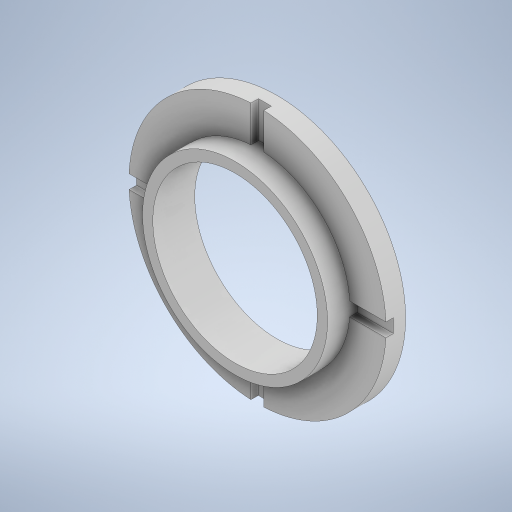
# Autodesk Inventor part: KY 58 Part
Saved by Autodesk Inventor 2024 (Build 280153000, 153)
## iProperties
Created: 2024-12-26
Part Number: KY 58 Part
Material: Generic
Document SubType Name: Modeling
Designer: Administrator
Density: 1 g/cm^3
Appearance: Default
Author: Administrator
Autodesk Inventor part; units mm, degrees
ref_plane "YZ Plane" through (0, 0, 0) normal (1, 0, 0) x (0, 1, 0)
ref_plane "XZ Plane" through (0, 0, 0) normal (0, 1, 0) x (-1, 0, 0)
ref_plane "XY Plane" through (0, 0, 0) normal (0, 0, 1) x (1, 0, 0)
sketch "Sketch1" plane through (0, 0, 0) normal (0, 0, 1) x (1, 0, 0)
  line L0 (-73.2799, 44.0426) -> (79.8189, 44.0426) construction
  line L1 (79.8189, 44.0426) -> (79.8189, -42.434) construction
  line L2 (79.8189, -42.434) -> (-73.2799, -42.434) construction
  line L3 (-73.2799, -42.434) -> (-73.2799, 44.0426) construction
  circle A0 centre (0.9241, -2.5998) radius 8.239
  circle A1 centre (0.9241, -2.5998) radius 12.8881
  point P0 (0, 0)
  constraints: 2 centre point, 2 other
extrude "Extrusion1" add sketch "Sketch1" along normal blind 1.2
sketch "Sketch2" plane through (0.9241, -2.5998, 1.2) normal (0, 0, 1) x (1, 0, 0)
  circle A0 centre (0, 0) radius 8.239 projected
  circle A1 centre (0, 0) radius 9.2643
  point P0 (-0.9241, 2.5998)
  constraints: 1 centre point
extrude "Extrusion2" add sketch "Sketch2" along normal blind 3
sketch "Sketch3" plane through (0.9241, -2.5998, 1.2) normal (0, 0, 1) x (1, 0, 0)
  circle A0 centre (0, 0) radius 9.1906
  arc A1 (12.8725, 0.6343) -> (0.6367, 12.8724) centre (0, 0) ccw
  arc A2 (-0.6581, 12.8713) -> (-12.8725, 0.6343) centre (0, 0) ccw
  arc A3 (-12.8667, -0.7427) -> (-0.6581, -12.8713) centre (0, 0) ccw
  arc A4 (0.6367, -12.8724) -> (12.8667, -0.7427) centre (0, 0) ccw
  line L0 (-12.8725, 0.6343) -> (-9.1687, 0.6343)
  line L1 (-9.1605, -0.7427) -> (-12.8667, -0.7427)
  line L2 (-0.6581, -12.8713) -> (-0.6581, -9.167)
  line L3 (0.6367, -9.1685) -> (0.6367, -12.8724)
  line L4 (12.8667, -0.7427) -> (9.1605, -0.7427)
  line L5 (9.1687, 0.6343) -> (12.8725, 0.6343)
  line L6 (0.6367, 12.8724) -> (0.6367, 9.1685)
  line L7 (-0.6581, 9.167) -> (-0.6581, 12.8713)
  point P0 (-0.9241, 2.5998)
  constraints: 16 end point, 8 parallel, 8 point on circle, 4 centre point, 1 coincident, 10 other
extrude "Extrusion3" add sketch "Sketch3" along normal blind 0.75 contours A0 L6 A1 L5 | L4 A4 L3 A0 | A0 L0 A2 L7 | L2 A3 L1 A0
sketch "Sketch4" plane through (0.9241, -2.5998, 0) normal (0, 0, -1) x (-1, 0, 0)
  circle A0 centre (-7.6761, 7.2071) radius 0.75
  circle A1 centre (0, 0) radius 8.239 projected
  circle A2 centre (-7.2071, -7.6761) radius 0.75
  circle A3 centre (7.6761, -7.2071) radius 0.75
  circle A4 centre (7.2071, 7.6761) radius 0.75
  point P0 (0.9241, 2.5998)
  dimension "d19" = 1.5
  dimension "d22" = 360
  constraints: 4 centre point, 9 other
  measures "d19" diameter of A0
extrude "Extrusion4" cut sketch "Sketch4" against normal blind 1.7 contours A0 | A2 | A3 | A4
body "Solid1"
